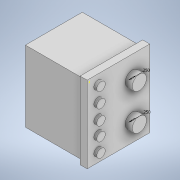
# Autodesk Inventor part: Battery 2
Saved by Autodesk Inventor 2022 (Build 260153000, 153)
## iProperties
Created: 2022-02-20
Part Number: Battery 2
Material: Generic
Document SubType Name: Modeling
Designer: kvaru
Density: 1 g/cm^3
Appearance: Default
Author: kvaru
Autodesk Inventor part; units mm, degrees
ref_plane "YZ Plane" through (0, 0, 0) normal (1, 0, 0) x (0, 1, 0)
ref_plane "XZ Plane" through (0, 0, 0) normal (0, 1, 0) x (-1, 0, 0)
ref_plane "XY Plane" through (0, 0, 0) normal (0, 0, 1) x (1, 0, 0)
sketch "Sketch1" plane through (0, 0, 0) normal (1, 0, 0) x (0, 1, 0)
  line L0 (0, 0) -> (-63.5, 0)
  line L1 (-63.5, 0) -> (-63.5, -50.8)
  line L2 (-63.5, -50.8) -> (0, -50.8)
  line L3 (0, -50.8) -> (0, 0)
  dimension "d0" = 63.5
  dimension "d1" = 50.8
  constraints: 8 end point, 2 parallel, 1 horizontal, 1 perpendicular
  measures "d0" distance of L2.end L1.end
  measures "d1" distance of L1.end L0.end
extrude "Extrusion1" add sketch "Sketch1" along normal blind 50.8
sketch "Sketch2" plane through (50.8, 0, 0) normal (1, 0, 0) x (0, 0, -1)
  line L0 (53.8638, 2.4661) -> (-2.0162, 2.4661)
  line L1 (-2.0162, 2.4661) -> (-2.0162, -66.1139)
  line L2 (-2.0162, -66.1139) -> (53.8638, -66.1139)
  line L3 (53.8638, -66.1139) -> (53.8638, 2.4661)
  point P0 (0, 0)
  dimension "d4" = 55.88
  dimension "d5" = 68.58
  constraints: 8 end point, 2 parallel, 1 horizontal, 1 perpendicular
  measures "d4" distance of L2.end L1.end
  measures "d5" distance of L1.end L0.end
extrude "Extrusion2" add sketch "Sketch2" along normal blind 6.35
sketch "Sketch3" plane through (57.15, 0, 0) normal (1, 0, 0) x (0, 0, -1)
  circle A0 centre (38.2887, -16.224) radius 6.35
  circle A1 centre (38.2887, -48.6721) radius 6.35
  circle A2 centre (6.879, -6.1002) radius 3.81
  circle A3 centre (6.879, -18.8199) radius 3.81
  circle A4 centre (6.879, -34.395) radius 3.81
  circle A5 centre (6.879, -46.5954) radius 3.81
  circle A6 centre (6.879, -58.7959) radius 3.81
  point P0 (0, 0)
  dimension "d8" = 12.7
  dimension "d9" = 12.7
  dimension "d10" = 7.62
  dimension "d11" = 7.62
  dimension "d12" = 7.62
  dimension "d13" = 7.62
  dimension "d14" = 7.62
  constraints: 7 centre point
  measures "d8" diameter of A0
  measures "d9" diameter of A1
  measures "d10" diameter of A2
  measures "d11" diameter of A3
  measures "d12" diameter of A4
  measures "d13" diameter of A5
  measures "d14" diameter of A6
extrude "Extrusion3" add sketch "Sketch3" along normal blind 6.35 contours A0 | A1
sketch "Sketch4" plane through (57.15, 0, 0) normal (1, 0, 0) x (0, 0, -1)
  circle A0 centre (7.7755, -6.0244) radius 3.81
  circle A1 centre (7.7755, -19.3217) radius 3.81
  circle A2 centre (7.7755, -32.619) radius 3.81
  circle A3 centre (7.7755, -44.7893) radius 3.81
  circle A4 centre (7.7755, -57.6359) radius 3.81
  point P0 (0, 0)
  dimension "d17" = 7.62
  dimension "d18" = 7.62
  dimension "d19" = 7.62
  dimension "d20" = 7.62
  dimension "d21" = 7.62
  constraints: 5 centre point
  measures "d17" diameter of A0
  measures "d18" diameter of A1
  measures "d19" diameter of A2
  measures "d20" diameter of A3
  measures "d21" diameter of A4
extrude "Extrusion4" add sketch "Sketch4" along normal blind 2.54
sketch "Sketch5" plane through (57.15, 0, 0) normal (1, 0, 0) x (0, 0, -1)
  point P0 (0, 0)
sketch "Sketch6" plane through (57.15, 0, 0) normal (1, 0, 0) x (0, 0, -1)
  circle A0 centre (38.3083, -15.968) radius 3.175
  circle A1 centre (38.3083, -48.6538) radius 3.175
  point P0 (0, 0)
  dimension "d24" = 6.35
  dimension "d25" = 6.35
  constraints: 2 centre point
  measures "d24" diameter of A0
  measures "d25" diameter of A1
body "Solid1"
